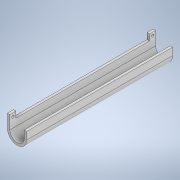
# Autodesk Inventor part: StraightTrack
Saved by Autodesk Inventor 2020 (Build 240168000, 168)
## iProperties
Created: 2020-02-20
Part Number: StraightTrack
Material: Generic
Document SubType Name: Modeling
Designer: brand
Density: 1 g/cm^3
Appearance: Default
Author: brand
Autodesk Inventor part; units mm, degrees
ref_plane "YZ Plane" through (0, 0, 0) normal (1, 0, 0) x (0, 1, 0)
ref_plane "XZ Plane" through (0, 0, 0) normal (0, 1, 0) x (-1, 0, 0)
ref_plane "XY Plane" through (0, 0, 0) normal (0, 0, 1) x (1, 0, 0)
sketch "Sketch1" plane through (0, 0, 0) normal (0, 0, 1) x (1, 0, 0)
  circle A0 centre (0, 0) radius 7.62
  line L0 (-10.16, 7.62) -> (-10.16, 0)
  arc A1 (-10.16, 0) -> (10.16, 0) centre (0, 0) ccw
  line L1 (10.16, 0) -> (10.16, 7.62)
  line L2 (10.16, 7.62) -> (7.62, 7.62)
  line L3 (7.62, 7.62) -> (7.62, 0)
  line L4 (-10.16, 7.62) -> (-7.62, 7.62)
  line L5 (-7.62, 7.62) -> (-7.62, 0)
  dimension "d0" = 15.24
  dimension "d1" = 2.54
  dimension "d2" = 2.54
  dimension "d3" = 2.54
  constraints: 12 end point, 4 point on circle, 2 centre point, 2 coincident, 2 tangent, 2 vertical, 1 horizontal, 1 point on line
  measures "d0" diameter of A0
  measures "d1" distance edge to line of A0 L0
  measures "d2" distance edge to line of A0 L1
  measures "d3" radial gap between concentric circles of A0 A1
extrude "Extrusion1" add sketch "Sketch1" along normal blind 152.4 contours L3 L2 L1 A1 L0 L4 L5 A0
sketch "Sketch2" plane through (-7.62, 0, 0) normal (1, 0, 0) x (0, 0, -1)
  line L0 (0, 7.62) -> (-152.4, 7.62) projected
  line L1 (0, 7.62) -> (-6.35, 7.62)
  line L2 (-6.35, 7.62) -> (-6.35, 13.97)
  line L3 (-6.35, 13.97) -> (0, 13.97)
  line L4 (0, 13.97) -> (0, 7.62)
  circle A0 centre (-3.175, 10.795) radius 1.27
  point P0 (0, 0)
  dimension "d6" = 6.35
  dimension "d7" = 6.35
  dimension "d8" = 2.54
  dimension "d9" = 3.175
  dimension "d10" = 3.175
  constraints: 8 end point, 2 parallel, 1 centre point, 1 horizontal, 1 perpendicular
  measures "d6" distance of L2.end L3.end
  measures "d7" distance of L1.end L2.end
  measures "d8" diameter of A0
  measures "d9" distance from line of L4 A0.centre
  measures "d10" distance from line of L0 A0.centre
extrude "Extrusion2" add sketch "Sketch2" against normal up to surface (2.54 mm away)
sketch "Sketch4" plane through (-7.62, 0, 152.4) normal (1, 0, 0) x (0, 0, -1)
  line L0 (0, 0) -> (0, 7.62) projected
  circle A0 centre (3.175, 10.473) radius 1.27
  line L1 (152.4, 7.62) -> (0, 7.62) projected
  line L2 (6.35, 7.62) -> (0, 7.62)
  line L3 (0, 7.62) -> (6.35, 7.62)
  line L4 (6.35, 7.62) -> (6.35, 13.97)
  line L5 (6.35, 13.97) -> (0, 13.97)
  line L6 (0, 13.97) -> (0, 7.62)
  point P0 (152.4, 0)
  dimension "d15" = 2.54
  dimension "d16" = 6.35
  dimension "d17" = 6.35
  constraints: 10 end point, 2 parallel, 1 centre point, 1 collinear, 1 horizontal, 1 perpendicular, 1 point on line
  measures "d15" diameter of A0
  measures "d16" distance of L5.end L4.end
  measures "d17" distance of L4.end L3.end
extrude "Extrusion3" add sketch "Sketch4" against normal up to surface (2.54 mm away)
body "Solid1"
